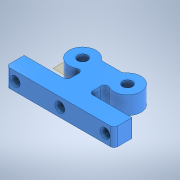
# Autodesk Inventor part: 4mm_Roller_Spacer
Saved by Autodesk Inventor 2021 (Build 250183000, 183)
## iProperties
Created: 2021-03-29
Part Number: 4mm_Roller_Spacer
Material: PET Plastic
Document SubType Name: Modeling
Designer: Jorian Brusind
Density: 1.541 g/cm^3
Appearance: Cyan
Author: Jorian Brusind
Autodesk Inventor part; units mm, degrees
ref_plane "YZ Plane" through (0, 0, 0) normal (1, 0, 0) x (0, 1, 0)
ref_plane "XZ Plane" through (0, 0, 0) normal (0, 1, 0) x (-1, 0, 0)
ref_plane "XY Plane" through (0, 0, 0) normal (0, 0, 1) x (1, 0, 0)
sketch "Sketch4" plane through (0, 0, 0) normal (0, 1, 0) x (-1, 0, 0)
  circle A0 centre (0, 0) radius 7.5
  circle A1 centre (0, 0) radius 2.75
  dimension "d19" = 15
  dimension "d20" = 5.5
  constraints: 2 centre point, 2 coincident
  measures "d19" diameter of A0
  measures "d20" diameter of A1
extrude "Extrusion4" add sketch "Sketch4" along normal blind 10
ref_plane "Work Plane2" through (0, 5, 0) normal (0, 1, 0) x (1, 0, 0)
sketch "Sketch12" plane through (0, 5, 0) normal (0, 1, 0) x (1, 0, 0)
  circle A0 centre (0, 0) radius 2.75 projected
  line L0 (0, 0) -> (25, 0)
  circle A1 centre (25, 0) radius 2.75
  circle A2 centre (25, 0) radius 7.5
  line L1 (12.5, 0) -> (12.5, -20)
  line L2 (42.5, -25) -> (-17.5, -25)
  line L3 (-17.5, -25) -> (-17.5, -15)
  line L4 (-17.5, -15) -> (42.5, -15)
  line L5 (42.5, -15) -> (42.5, -25)
  line L6 (42.5, -25) -> (-17.5, -15) construction
  line L7 (-17.5, -25) -> (42.5, -15) construction
  circle A3 centre (0, 0) radius 7.5 projected
  line L8 (18.6557, -4) -> (6.3443, -4)
  line L9 (6.3443, -4) -> (6.3443, 4)
  line L10 (6.3443, 4) -> (18.6557, 4)
  line L11 (18.6557, 4) -> (18.6557, -4)
  line L12 (18.6557, -4) -> (6.3443, 4) construction
  line L13 (6.3443, -4) -> (18.6557, 4) construction
  line L14 (6.3443, 4) -> (18.6557, 4)
  line L15 (18.6557, 4) -> (18.6557, -16)
  line L16 (18.6557, -16) -> (6.3443, -16)
  line L17 (6.3443, -16) -> (6.3443, 4)
  point P0 (6.3443, -15)
  point P1 (18.6557, -15)
  dimension "d66" = 25
  dimension "d67" = 5.5
  dimension "d68" = 15
  dimension "d69" = 20
  dimension "d70" = 60
  dimension "d71" = 10
  dimension "d72" = 8
  dimension "d73" = 20
  constraints: 36 end point, 6 parallel, 5 midpoint, 4 horizontal, 3 perpendicular, 2 centre point, 2 coincident, 1 vertical, 2 other
  measures "d66" distance of L0.start L0.end
  measures "d67" diameter of A1
  measures "d68" diameter of A2
  measures "d69" distance of L1.start L1.end
  measures "d70" distance of L3.end L4.end
  measures "d71" distance of L2.end L3.end
  measures "d72" distance of L8.end L9.end
  measures "d73" distance of L14.end L15.end
extrude "Extrusion10" add sketch "Sketch12" along normal mid plane 10 contours A3 L10 A2 L0 | L0 L1 L8 A3 | L0 A2 L8 L1 | L8 L1 L4 L17 | A2 L11 L0 | L0 L11 A2 | L8 L15 L4 L1 | A2 L11 | L17 L16 L15 L4 L5 L2 L3 | L4 L1 L16 L17 | L4 L15 L16 L1
sketch "Sketch13" plane through (18.6557, 10, -4) normal (0, 0, -1) x (-1, 0, 0)
  line L0 (0, 0) -> (12.3114, 0) projected
  line L1 (6.1557, 0) -> (6.1557, -5)
  line L2 (6.1557, -9.6188) -> (2.1557, -7.3094)
  line L3 (2.1557, -7.3094) -> (2.1557, -2.6906)
  line L4 (2.1557, -2.6906) -> (6.1557, -0.3812)
  line L5 (6.1557, -0.3812) -> (10.1557, -2.6906)
  line L6 (10.1557, -2.6906) -> (10.1557, -7.3094)
  line L7 (10.1557, -7.3094) -> (6.1557, -9.6188)
  line L8 (36.1557, -10) -> (36.1557, 0) projected
  line L9 (36.1557, -5) -> (31.1557, -5)
  line L10 (31.1557, -9.6188) -> (27.1557, -7.3094)
  line L11 (27.1557, -7.3094) -> (27.1557, -2.6906)
  line L12 (27.1557, -2.6906) -> (31.1557, -0.3812)
  line L13 (31.1557, -0.3812) -> (35.1557, -2.6906)
  line L14 (35.1557, -2.6906) -> (35.1557, -7.3094)
  line L15 (35.1557, -7.3094) -> (31.1557, -9.6188)
  line L16 (-23.8443, -10) -> (-23.8443, 0) projected
  line L17 (-23.8443, -5) -> (-18.8443, -5)
  line L18 (-23.8443, -5) -> (-18.8443, -5) construction
  line L19 (-18.8443, -9.6188) -> (-22.8443, -7.3094)
  line L20 (-22.8443, -7.3094) -> (-22.8443, -2.6906)
  line L21 (-22.8443, -2.6906) -> (-18.8443, -0.3812)
  line L22 (-18.8443, -0.3812) -> (-14.8443, -2.6906)
  line L23 (-14.8443, -2.6906) -> (-14.8443, -7.3094)
  line L24 (-14.8443, -7.3094) -> (-18.8443, -9.6188)
  point P0 (18.6557, -10)
  dimension "d76" = 5
  dimension "d77" = 8
  dimension "d78" = 5
  dimension "d79" = 8
  dimension "d80" = 5
  dimension "d81" = 0
  dimension "d82" = 8
  constraints: 44 end point, 3 coincident, 3 horizontal, 3 midpoint, 3 parallel, 1 collinear, 1 vertical, 39 other
  measures "d76" distance of L1.start L1.end
  measures "d77" distance between parallel lines of L3 L6
  measures "d78" distance of L9.start L9.end
  measures "d79" distance between parallel lines of L11 L14
  measures "d80" distance of L17.start L17.end
  measures "d81" distance between parallel lines of L17 L18
  measures "d82" distance between parallel lines of L20 L23
extrude "Extrusion11" cut sketch "Sketch13" against normal blind 23
fillet "Fillet4" radius 2 8 edges at (18.6557, 5, 15) (6.3443, 5, 15) (-17.5, 5, 25) (42.5, 5, 25) (6.3443, 5, -4) (18.6557, 5, -4) (18.6557, 5, 4) (6.3443, 5, 4)
sketch "Sketch14" plane through (17.6345, 0, -4) normal (0, 0, -1) x (-1, 0, 0)
  circle A0 centre (5.2691, 5) radius 2.75
  line L0 (0, 10) -> (10.2691, 10) projected
  line L1 (10.2691, 10) -> (10.2691, 0) projected
  circle A1 centre (-19.8655, 5) radius 2.75
  circle A2 centre (30.1345, 5) radius 2.75
  line L2 (35.1345, 0) -> (35.1345, 10) projected
  line L3 (-24.8655, 0) -> (-24.8655, 10) projected
  point P0 (17.6345, 0)
  dimension "d86" = 5.5
  dimension "d87" = 5
  dimension "d88" = 5
  dimension "d89" = 5.5
  dimension "d90" = 5.5
  dimension "d91" = 5
  dimension "d92" = 5
  constraints: 3 centre point, 2 horizontal alignment
  measures "d86" diameter of A0
  measures "d87" distance from line of L0 A0.centre
  measures "d88" distance from line of L1 A0.centre
  measures "d89" diameter of A1
  measures "d90" diameter of A2
  measures "d91" distance from line of L2 A2.centre
  measures "d92" distance from line of L3 A1.centre
extrude "Extrusion12" cut sketch "Sketch14" against normal through all
body "Solid2"
